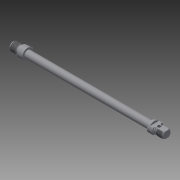
# Autodesk Inventor part: 19197 DSNU-12-200-P---(A----0-ZR)
Saved by Autodesk Inventor 2014 SP2 (Build 180246200, 246)
## iProperties
Created: 2019-05-10
Part Number: 19197 DSNU-12-200-P---(A----0-ZR)
Material: Generic
Catalog Web Link: www.cadenas.de
Description: DSNU---(ZR)-Standard cylinder
Vendor: FESTO
Document SubType Name: Modeling
Designer: psadmin
Manufacturer: FESTO
Mass: 19.1949 g
Surface Area: 224.329 cm^2
Volume: 19.1949 cm^3
Density: 1 g/cm^3
Appearance: PSOLRGB-192-192-192
Category: PARTsolutions
Company: FESTO
Title: 19197 DSNU-12-200-P
Author: Cadenas PARTsolutions
Comments: Standard cylinder
PSOL_IDENT_0: {$CADENAS_DATA\23d-libs\festo\parts\d\dsnu\parts\dsnu_metric_zr.prj},234 {VTYP=3D},{NB=19197 DSNU-12
PSOL_IDENT_1: -200-P---(A----0-ZR)},{LINA=19197 DSNU-12-200-P},{NN=DSNU---(ZR)},{DATE=02.05.2019 17:52:25},{GEOMDA
PSOL_IDENT_2: TE=09.08.2018 14:24:00},{VERSION=},{LINEID=30},{WBVAR=TNR,HUB,DA,PE,ZD,VS,KA,K8,KP,R8},{WBNUMERIC=HU
PSOL_IDENT_3: B,K8}  {NB=19197 DSNU-12-200-P---(A----0-ZR)},{LINA=19197 DSNU-12-200-P},{KT=DUMMY},{TNR=19197},{TYP=
PSOL_IDENT_4: DSNU-12},{DSNU=METRIC},{DE=D},{KDM=12},{HUB=200},{DA=P},{DA1='P','PPV'},{PE=A},{ZD=-},{VS=-},{VSALG='
PSOL_IDENT_5: -','Q'},{KA=-},{KAALG='-','S2'},{K8=0},{KP=-},{KPALG='-','KP'},{R8=-},{R81='-'},{R8H=0.000},{A1=20},
PSOL_IDENT_6: {A2=100},{A3=4},{A4=38.0},{AB=16},{AM=16},{B=16},{BB=3},{BE=M16x1,5},{BENDM=16.000},{BEKDM=14.160},{
PSOL_IDENT_7: BEP=1.500},{BS=4.5},{B1=30},{B2=0},{B3=0},{B4=0},{B5=18.1},{B6=8},{B7=0},{CD=6},{D=20},{D1=16},{D2=6
PSOL_IDENT_8: },{D3=13.3},{D4=5.5},{D5=14.5},{D6=0},{D7=0},{EE=M5},{EENDM=5.0000},{EEKDM=4.0190},{EW=12},{F=23},{F
PSOL_IDENT_9: F=M4},{FFNDM=4.000},{FFKDM=3.141},{F1=0},{H=22},{H1=0},{KK=M6},{KKNDM=6.0000},{KKKDM=4.7730},{KKP=0.
PSOL_IDENT_10: 000},{K1=-},{K1NDM=0.000},{K1KDM=0.000},{K2=0.0},{KV=24},{KW=8},{L=9},{LH=6.0},{LK=7.7},{L1=89},{L2=
PSOL_IDENT_11: 50},{L3=6.0},{L4=17.0},{L5=15},{L6=38},{L7=21},{L8=10.0},{L9=23.0},{L10=61.8},{L11=71.8},{L12=47.7},
PSOL_IDENT_12: {L13=94.0},{ST=4.5},{SW=5},{T=0},{WH=22},{X=0.0},{XC=75},{K1KP=32},{K2KP=M5},{K2KPNDM=5.000},{K3KP=1
PSOL_IDENT_13: 1},{K4KP=16.0},{K5KP=41.0},{K6KP=4.2},{K7KP=16},{K8KP=24.0},{K9KP=10.0},{K10KP=0.0},{K11KP=0},{K12KP=
PSOL_IDENT_14: M5},{K12KPNDM=5.000},{K13KP=38},{ZRSTART=27},{MHL=21.800},{ZRL=30},{C=9.500},{WHX=10.000},{LD1=14.00
PSOL_IDENT_15: 0},{LD2=13.700},{AD1=7.000},{AD2=5.000},{AD3=11.000},{AD4=6.000},{AD5=0.000},{MH1=9.000},{MH2=3.200}
PSOL_IDENT_16: ,{MH3=12.000},{KP1=22.500},{KP2=12.000},{KP3=9.600},{KP4=15.000},{KP5=20.000},{KPC=14.000},{KPF=3.00
PSOL_IDENT_17: 0},{KPG=10.000},{KPH=35.000},{KPJ=15.500},{KPK=11.000},{KPL=2.500},{KPR3=0.800},{KPR=15.000},{KPS=8.
PSOL_IDENT_18: 500},{MLD1=30.000},{MLD2=24.000},{MLD3=4.000},{MLL1=10.000},{PPVSTD=6.000},{PPVMH=18.100},{PPVMQ=1.8
PSOL_IDENT_19: 50},{PPVY=7.500},{PPVZ=5.700},{PPVA=3.000},{PPVB=0.200},{PPVC=0.600},{PPVD=0.700},{PPVE=3.200},{PPVH=
PSOL_IDENT_20: 11.000},{KL1=42.3},{SWL=3.000},{K3L=0.000},{ES1=1.000},{ES2=0.000},{KPVERS=0},{HUB1=200},{NUTOFF=8.0
PSOL_IDENT_21: 00},{DIMZJREAR=284},{KAVERS=0},{VERS=1},{H2=18}
NN: DSNU---(ZR)
NT: Standard cylinder
NB: 19197 DSNU-12-200-P---(A----0-ZR)
NBSYN: $TNR. $TYP.-$HUB1.-$DA.---($PE.$ZD.$VS.$KA.$KP.$K8.$R8.ZR)
LINA: 19197 DSNU-12-200-P
TNR: 19197
TYP: DSNU-12
DSNU: METRIC
DE: D
KDM: 12
HUB: 200
DA: P
DA1: 'P','PPV'
PE: A
ZD: -
VS: -
KA: -
K8: 0
KP: -
R8: -
R81: '-'
R8H: 0
A1: 20
A2: 100
A3: 4
A4: 38
AB: 16
AM: 16
B: 16
BB: 3
BE: M16x1,5
BENDM: 16
BEKDM: 14.16
BEP: 1.5
BS: 4.5
B1: 30
B2: 0
B3: 0
B4: 0
B5: 18.1
B6: 8
B7: 0
CD: 6
D: 20
D1: 16
D2: 6
D3: 13.3
D4: 5.5
D5: 14.5
D6: 0
D7: 0
EE: M5
EENDM: 5
EEKDM: 4.019
EW: 12
F: 23
FF: M4
FFNDM: 4
FFKDM: 3.141
F1: 0
H: 22
H1: 0
KK: M6
KKNDM: 6
KKKDM: 4.773
KKP: 0
K1: -
K1NDM: 0
K1KDM: 0
K2: 0
KV: 24
KW: 8
L: 9
LH: 6
LK: 7.7
L3: 6
L4: 17
L5: 15
L6: 38
L7: 21
L8: 10
L9: 23
L13: 94
ST: 4.5
SW: 5
T: 0
X: 0
K1KP: 32
K2KP: M5
K2KPNDM: 5
K3KP: 11
K4KP: 16
K5KP: 41
K6KP: 4.2
K7KP: 16
K8KP: 24
K9KP: 10
K10KP: 0
K11KP: 0
K12KP: M5
K12KPNDM: 5
K13KP: 38
MHL: 21.8
C: 9.5
WHX: 10
LD1: 14
LD2: 13.7
AD1: 7
AD2: 5
AD3: 11
AD4: 6
AD5: 0
MH1: 9
MH2: 3.2
MH3: 12
KP1: 22.5
KP2: 12
KP3: 9.6
KP4: 15
KP5: 20
KPC: 14
KPF: 3
KPG: 10
KPH: 35
KPJ: 15.5
KPK: 11
KPL: 2.5
KPR3: 0.8
KPR: 15
KPS: 8.5
MLD1: 30
MLD2: 24
MLD3: 4
MLL1: 10
PPVSTD: 6
PPVMH: 18.1
PPVMQ: 1.85
PPVY: 7.5
PPVZ: 5.7
PPVA: 3
PPVB: 0.2
PPVC: 0.6
PPVD: 0.7
PPVE: 3.2
PPVH: 11
SWL: 3
K3L: 0
ES1: 1
ES2: 0
NUTOFF: 8
H2: 18
SUPPLIER: FESTO
ARTICLENO: 19197 DSNU-12-200-P---(A----0-ZR)
BOMINFO: 19197 DSNU-12-200-P
CREATOR: CADENAS GmbH
Autodesk Inventor part; units mm, degrees
ref_plane "YZ Plane" through (0, 0, 0) normal (1, 0, 0) x (0, 1, 0)
ref_plane "XZ Plane" through (0, 0, 0) normal (0, 1, 0) x (-1, 0, 0)
ref_plane "XY Plane" through (0, 0, 0) normal (0, 0, 1) x (1, 0, 0)
sketch "Sketch_1" plane through (0, 0, 0) normal (0, 0, 1) x (1, 0, 0)
  line L0 (17, 0) -> (0, 0)
  line L1 (0, 0) -> (0, 6.8)
  line L2 (0, 6.8) -> (0.2, 7)
  line L3 (0.2, 7) -> (1, 7)
  line L4 (1, 7) -> (2, 8)
  line L5 (2, 8) -> (11.95, 8)
  line L6 (11.95, 8) -> (12.8657, 7.0843)
  arc A0 (12.8657, 7.0843) -> (13.4314, 6.85) centre (13.4314, 7.65) ccw
  line L7 (13.4314, 6.85) -> (14.2, 6.85)
  arc A1 (14.2, 6.85) -> (15, 7.65) centre (14.2, 7.65) ccw
  line L8 (15, 7.65) -> (15, 8)
  line L9 (15, 8) -> (17, 8)
  line L10 (17, 8) -> (17, 0)
  line L11 (17, 0) -> (0, 0)
  constraints: 24 end point, 4 point on circle, 2 centre point
revolve "Revolution1" add sketch "Sketch_1" angle 360 about axis through (17, 0, 0) along (1, 0, 0)
thread "Thread1" size "M16x1.5" class "6g" standard "ISO Metric profile" full length
sketch "Sketch_2" plane through (17, 0, 0) normal (1, 0, 0) x (0, 0, -1)
  arc A0 (-4.9029, 8.7156) -> (4.9029, 8.7156) centre (0, 0) ccw
  arc A1 (4.75, 8.9771) -> (4.9029, 8.7156) centre (5.05, 8.9771) ccw
  line L0 (4.75, 8.9771) -> (4.75, 9.6)
  arc A2 (4.75, 9.6) -> (4.35, 10) centre (4.35, 9.6) ccw
  line L1 (4.35, 10) -> (-4.35, 10)
  arc A3 (-4.35, 10) -> (-4.75, 9.6) centre (-4.35, 9.6) ccw
  line L2 (-4.75, 9.6) -> (-4.75, 8.9771)
  arc A4 (-4.9029, 8.7156) -> (-4.75, 8.9771) centre (-5.05, 8.9771) ccw
  constraints: 10 point on circle, 6 end point, 5 centre point
extrude "Extrusion1" add sketch "Sketch_2" along normal blind 10
sketch "Sketch_3" plane through (0, 0, 0) normal (0, 0, 1) x (1, 0, 0)
  line L0 (257, 0) -> (27, 0)
  line L1 (27, 0) -> (27, 6.65)
  line L2 (27, 6.65) -> (257, 6.65)
  line L3 (257, 6.65) -> (257, 0)
  line L4 (257, 0) -> (27, 0)
  constraints: 10 end point
revolve "Revolution2" add sketch "Sketch_3" angle 360 about axis through (257, 0, 0) along (1, 0, 0)
sketch "Sketch_16" plane through (257, 0, 0) normal (1, 0, 0) x (0, 0, -1)
  arc A0 (-4.9029, 8.7156) -> (4.9029, 8.7156) centre (0, 0) ccw
  arc A1 (4.75, 8.9771) -> (4.9029, 8.7156) centre (5.05, 8.9771) ccw
  line L0 (4.75, 8.9771) -> (4.75, 9.6)
  arc A2 (4.75, 9.6) -> (4.35, 10) centre (4.35, 9.6) ccw
  line L1 (4.35, 10) -> (-4.35, 10)
  arc A3 (-4.35, 10) -> (-4.75, 9.6) centre (-4.35, 9.6) ccw
  line L2 (-4.75, 9.6) -> (-4.75, 8.9771)
  arc A4 (-4.9029, 8.7156) -> (-4.75, 8.9771) centre (-5.05, 8.9771) ccw
  constraints: 10 point on circle, 6 end point, 5 centre point
extrude "Extrusion2" add sketch "Sketch_16" along normal blind 10
sketch "Sketch_23" plane through (0, 0, 0) normal (0, 0, 1) x (1, 0, 0)
  line L0 (284, 0) -> (267, 0)
  line L1 (267, 0) -> (267, 8)
  line L2 (267, 8) -> (269, 8)
  line L3 (269, 8) -> (269, 7.65)
  arc A0 (269, 7.65) -> (269.8, 6.85) centre (269.8, 7.65) ccw
  line L4 (269.8, 6.85) -> (270.5686, 6.85)
  arc A1 (270.5686, 6.85) -> (271.1343, 7.0843) centre (270.5686, 7.65) ccw
  line L5 (271.1343, 7.0843) -> (272.05, 8)
  line L6 (272.05, 8) -> (282, 8)
  line L7 (282, 8) -> (283, 7)
  line L8 (283, 7) -> (283.8, 7)
  line L9 (283.8, 7) -> (284, 6.8)
  line L10 (284, 6.8) -> (284, 0)
  line L11 (284, 0) -> (267, 0)
  constraints: 24 end point, 4 point on circle, 2 centre point
revolve "Revolution3" add sketch "Sketch_23" angle 360 about axis through (284, 0, 0) along (1, 0, 0)
thread "Thread2" size "M16x1.5" class "6g" standard "ISO Metric profile" full length
sketch "Sketch_6" plane through (0, 0, 0) normal (0, 1, 0) x (-1, 0, 0)
  line L0 (-261, -18) -> (-261, -6)
  line L1 (-261, -6) -> (-284, -6)
  line L2 (-284, -6) -> (-284, 6)
  line L3 (-284, 6) -> (-261, 6)
  line L4 (-261, 6) -> (-261, 18)
  line L5 (-261, 18) -> (-296, 18)
  line L6 (-296, 18) -> (-296, -18)
  line L7 (-296, -18) -> (-261, -18)
  constraints: 16 end point
extrude "Extrusion3" cut sketch "Sketch_6" along normal mid plane 20
sketch "Sketch7" plane through (282, -5.2915, -6) normal (0, 0, -1) x (-1, 0, 0)
  point P0 (12, 5.2915)
hole "Hole1" at (270, 0, -6) direction (0, 0, 1) diameter 6 depth 12
sketch "Sketch8" plane through (17, 10, 4.35) normal (0, 1, 0) x (1, 0, 0)
  point P0 (6, 4.35)
hole "Hole2" at (23, 10, 0) direction (0, -1, 0) diameter 4.134 depth 10 countersink diameter 5 countersink angle 90 thread size "M5x0.8" class "6H" standard "ISO Metric profile"
sketch "Sketch9" plane through (257, 10, 4.35) normal (0, 1, 0) x (1, 0, 0)
  point P0 (4, 4.35)
hole "Hole3" at (261, 10, 0) direction (0, -1, 0) diameter 4.134 depth 11 tip angle 120 countersink diameter 5 countersink angle 90 thread size "M5x0.8" class "6H" standard "ISO Metric profile"
sketch "Sketch_64" plane through (0, 0, 0) normal (0, 0, 1) x (1, 0, 0)
  line L0 (240.3, 0) -> (-5, 0)
  line L1 (-5, 0) -> (-5, 3)
  line L2 (-5, 3) -> (37.3, 3)
  line L3 (37.3, 3) -> (37.3, 6)
  line L4 (37.3, 6) -> (240.3, 6)
  line L5 (240.3, 6) -> (240.3, 0)
  line L6 (240.3, 0) -> (-5, 0)
  constraints: 14 end point
revolve "Revolution4" cut sketch "Sketch_64" angle 360 about axis through (240.3, 0, 0) along (1, 0, 0)
ref_plane "FDT_FRONT_XY" through (17, 0, 0) normal (1, 0, 0) x (0, 0, -1)
ref_plane "FDT_FRONT_YZ" through (17, 0, 0) normal (0, 0, -1) x (0, 1, 0)
ref_plane "FDT_FRONT_ZX" through (17, 0, 0) normal (0, 1, 0) x (1, 0, 0)
ref_plane "FDT_QSFRONT_XY" through (23, 10, 0) normal (0, 1, 0) x (0, 0, 1)
ref_plane "FDT_QSFRONT_YZ" through (23, 10, 0) normal (0, 0, 1) x (1, 0, 0)
ref_plane "FDT_QSFRONT_ZX" through (23, 10, 0) normal (1, 0, 0) x (0, 1, 0)
ref_plane "FDT_QSREAR_XY" through (261, 10, 0) normal (0, 1, 0) x (0, 0, 1)
ref_plane "FDT_QSREAR_YZ" through (261, 10, 0) normal (0, 0, 1) x (1, 0, 0)
ref_plane "FDT_QSREAR_ZX" through (261, 10, 0) normal (1, 0, 0) x (0, 1, 0)
ref_plane "FDT_REAR_XY" through (267, 0, 0) normal (-1, 0, 0) x (0, 0, -1)
ref_plane "FDT_REAR_YZ" through (267, 0, 0) normal (0, 0, -1) x (0, -1, 0)
ref_plane "FDT_REAR_ZX" through (267, 0, 0) normal (0, -1, 0) x (-1, 0, 0)
ref_plane "FDT_SMBR1_XY" through (36.5, 0, 0) normal (-1, 0, 0) x (0, 0, 1)
ref_plane "FDT_SMBR1_YZ" through (36.5, 0, 0) normal (0, 0, 1) x (0, 1, 0)
ref_plane "FDT_SMBR1_ZX" through (36.5, 0, 0) normal (0, 1, 0) x (-1, 0, 0)
ref_plane "FDT_SMBR2_XY" through (247.5, 0, 0) normal (-1, 0, 0) x (0, 0, 1)
ref_plane "FDT_SMBR2_YZ" through (247.5, 0, 0) normal (0, 0, 1) x (0, 1, 0)
ref_plane "FDT_SMBR2_ZX" through (247.5, 0, 0) normal (0, 1, 0) x (-1, 0, 0)
ref_plane "FDT_SWIVELAXIS_XY" through (270, 0, 0) normal (0, 0, 1) x (1, 0, 0)
ref_plane "FDT_SWIVELAXIS_YZ" through (270, 0, 0) normal (1, 0, 0) x (0, 1, 0)
ref_plane "FDT_SWIVELAXIS_ZX" through (270, 0, 0) normal (0, 1, 0) x (0, 0, 1)
ref_plane "NUT_XY" through (8, 0, 0) normal (1, 0, 0) x (0, 0, -1)
ref_plane "NUT_YZ" through (8, 0, 0) normal (0, 0, -1) x (0, 1, 0)
ref_plane "NUT_ZX" through (8, 0, 0) normal (0, 1, 0) x (1, 0, 0)
ref_plane "ZR_XY" through (0, 0, 0) normal (1, 0, 0) x (0, 0, -1)
ref_plane "ZR_YZ" through (0, 0, 0) normal (0, 0, -1) x (0, 1, 0)
ref_plane "ZR_ZX" through (0, 0, 0) normal (0, 1, 0) x (1, 0, 0)
ref_plane "ZYL_XY" through (17, 0, 0) normal (1, 0, 0) x (0, 0, -1)
ref_plane "ZYL_YZ" through (17, 0, 0) normal (0, 0, -1) x (0, 1, 0)
ref_plane "ZYL_ZX" through (17, 0, 0) normal (0, 1, 0) x (1, 0, 0)
body "Solid1"
